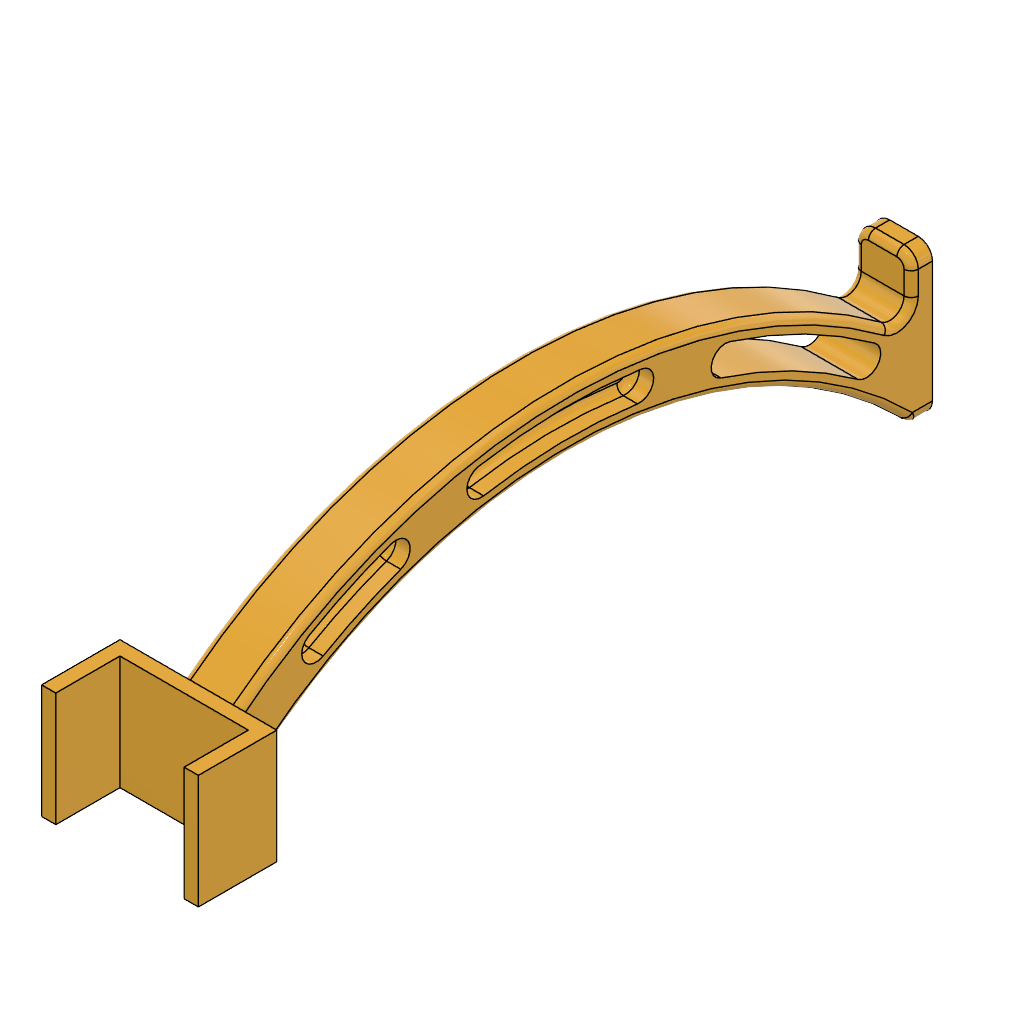
5. Marmik Shah_2026A4PS0775H - Landing Gear_Optimization study (Autodesk Fusion 360 design; units mm, degrees)
description: CATIA V5 STEP Exchange
part number: Landing stick.1.3
Autodesk Fusion 360 part; units mm, degrees
sketch "Sketch7" plane through (0, 0, 0) normal (0, 0, 1) x (1, 0, 0)
  line L0 (-11, 11) -> (11, 11)
  line L1 (11, 11) -> (11, -5)
  line L2 (11, -5) -> (-11, -5)
  line L3 (-11, -5) -> (-11, 11)
  dimension "d5" = 22
  dimension "d6" = 11
  dimension "d7" = 16
  dimension "d8" = 11
  constraint horizontal L0
  constraint vertical L1
  constraint horizontal L2
  constraint vertical L3
  measures "d5" distance of L0.start L0.end
  measures "d6" distance of origin L3
  measures "d7" distance of L0 L2
  measures "d8" distance of origin L0
extrude "Extrude1" add sketch "Sketch7" against normal blind 2
sketch "Sketch8" plane through (0, 0, 0) normal (1, 0, 0) x (0, 0, -1)
  arc A0 (98, 7.6281) -> (2, 7.6281) centre (50, -50) ccw
  arc A1 (98.7134, -4) -> (2, -3.256) centre (50, -50) ccw
  line L0 (98.7134, -4) -> (101, -4)
  line L1 (101, -4) -> (101, 17)
  line L2 (101, 17) -> (98, 17)
  line L3 (98, 17) -> (98, 7.6281)
  line L4 (2, -3.256) -> (2, 7.6281)
  dimension "d13" = 75
  dimension "d19" = 3
  dimension "d20" = 21
  dimension "d21" = 50
  dimension "d22" = 50
  dimension "d23" = 17
  dimension "d26" = 67
  dimension "d28" = 8
  dimension "d30" = 2
  dimension "d31" = 101
  constraint horizontal L0
  constraint vertical L1
  constraint horizontal L2
  constraint vertical L3
  constraint vertical A0.centre A1.centre
  constraint coincident A0.centre A1.centre
  constraint vertical L4
  measures "d13" radius of A0
  measures "d19" distance of L1 L3
  measures "d20" distance of L0.end L1.end
  measures "d21" horizontal distance of origin A0.centre
  measures "d22" vertical distance of origin A0.centre
  measures "d23" distance of origin L2
  measures "d26" radius of A1
  measures "d28" distance of A0 A1
  measures "d30" distance of origin L4
  measures "d31" distance of origin L1
extrude "Extrude3" add sketch "Sketch8" along normal blind 4 and the other way blind 4
sketch "Sketch11" plane through (0, 0, 0) normal (0, 0, 1) x (1, 0, 0)
  line L0 (-11, -5) -> (11, -5)
  line L1 (11, -5) -> (11, 11)
  line L2 (11, 11) -> (-11, 11)
  line L3 (-11, 11) -> (-11, -5)
  line L4 (11, -5) -> (9, -5)
  line L5 (9, -5) -> (9, 11)
  line L6 (9, 11) -> (11, 11)
  line L7 (11, 11) -> (11, -5)
  line L8 (-11, -5) -> (-9, -5)
  line L9 (-9, -5) -> (-9, 11)
  line L10 (-9, 11) -> (-11, 11)
  line L11 (-11, 11) -> (-11, -5)
  dimension "d84" = 2
  dimension "d85" = 2
  constraint coincident L0.start L3.end
  constraint horizontal L4
  constraint vertical L5
  constraint horizontal L6
  constraint vertical L7
  constraint horizontal L8
  constraint vertical L9
  constraint horizontal L10
  constraint vertical L11
  constraint horizontal L4.end L8.end
  constraint horizontal L5.end L9.end
  constraint coincident L2 L9.end
  constraint coincident L1.end L7
  measures "d84" distance of L5 L7
  measures "d85" distance of L9 L11
sketch "Sketch12" plane through (4, 0, 0) normal (1, 0, 0) x (0, 0, -1)
  line L0 (98.7134, -4) -> (101, -4)
  line L1 (101, -4) -> (101, 17)
  line L2 (101, 17) -> (98, 17)
  line L3 (98, 17) -> (98, 7.6281)
  arc A0 (98, 7.6281) -> (2, 7.6281) centre (50, -50) ccw
  line L4 (2, 7.6281) -> (2, -3.256)
  arc A1 (98.7134, -4) -> (2, -3.256) centre (50, -50) ccw
  arc A2 (98, 7.6281) -> (2, 7.6281) centre (50, -50) ccw
  arc A3 (25.0325, 18.5976) -> (13.5, 13.2199) centre (50, -50) ccw
  arc A4 (26.4006, 14.8388) -> (15.5, 9.7558) centre (50, -50) ccw
  arc A5 (13.5, 13.2199) -> (15.5, 9.7558) centre (14.5, 11.4878) ccw
  arc A6 (26.4006, 14.8388) -> (25.0325, 18.5976) centre (25.7166, 16.7182) ccw
  line L5 (50, -50) -> (14.5, 11.4878) construction
  line L6 (50, -50) -> (25.7166, 16.7182) construction
  line L7 (50, -50) -> (14.0011, -50) construction
  arc A7 (60.1596, 22.2896) -> (37.3237, 21.891) centre (50, -50) ccw
  arc A8 (59.6029, 18.3285) -> (38.0183, 17.9517) centre (50, -50) ccw
  arc A9 (37.3237, 21.891) -> (38.0183, 17.9517) centre (37.671, 19.9214) ccw
  arc A10 (59.6029, 18.3285) -> (60.1596, 22.2896) centre (59.8813, 20.309) ccw
  line L8 (50, -50) -> (37.671, 19.9214) construction
  line L9 (50, -50) -> (59.8813, 20.309) construction
  arc A11 (92.9083, 9.0582) -> (72.5582, 19.4271) centre (50, -50) ccw
  arc A12 (90.5572, 5.8222) -> (71.3222, 15.6229) centre (50, -50) ccw
  arc A13 (72.5582, 19.4271) -> (71.3222, 15.6229) centre (71.9402, 17.525) ccw
  arc A14 (90.5572, 5.8222) -> (92.9083, 9.0582) centre (91.7328, 7.4402) ccw
  line L10 (50, -50) -> (71.9402, 17.525) construction
  line L11 (50, -50) -> (91.7328, 7.4402) construction
  dimension "d46" = 73
  dimension "d47" = 4
  dimension "d48" = 2
  dimension "d49" = 2
  dimension "d50" = 10
  dimension "d51" = 60
  dimension "d54" = 73
  dimension "d55" = 4
  dimension "d56" = 2
  dimension "d57" = 2
  dimension "d58" = 18
  dimension "d59" = 10
  dimension "d60" = 73
  dimension "d61" = 4
  dimension "d62" = 2
  dimension "d63" = 2
  dimension "d64" = 18
  dimension "d65" = 10
  constraint coincident A0.centre A1.centre
  constraint tangent A3 A5
  constraint tangent A3 A6
  constraint coincident A5.centre L5.end
  constraint coincident A6.centre L6.end
  constraint horizontal L7
  constraint tangent A7 A9
  constraint tangent A7 A10
  constraint coincident A9.centre L8.end
  constraint coincident A10.centre L9.end
  constraint tangent A12 A13
  constraint tangent A12 A14
  constraint coincident A13.centre L10.end
  constraint coincident A14.centre L11.end
  measures "d46" radius of A3
  measures "d47" distance of A3 A4
  measures "d48" radius of A5
  measures "d49" radius of A6
  measures "d50" angle of L5 L6
  measures "d51" angle of L5 L7
  measures "d54" radius of A7
  measures "d55" distance of A7 A8
  measures "d56" radius of A10
  measures "d57" radius of A9
  measures "d58" angle of L8 L9
  measures "d59" angle of L6 L8
  measures "d60" radius of A11
  measures "d61" distance of A11 A12
  measures "d62" radius of A13
  measures "d63" radius of A14
  measures "d64" angle of L10 L11
  measures "d65" angle of L9 L10
extrude "Extrude5" cut sketch "Sketch12" against normal blind 3 contours A3 A4 A5 A6 | A7 A8 A9 A10
mirror "Mirror1" about plane through (0, 0, 0) normal (1, 0, 0) of "Extrude5"
fillet "Fillet6" radius 2 1 edges at (0, 7.6281, -98)
extrude "Extrude6" add sketch "Sketch11" along normal blind 9 contours L0 L2 L3 L8 L9 L10 L11 | L0 L1 L2 L4 L5 L6 L7
extrude "Extrude7" cut sketch "Sketch12" against normal up to surface (8 mm away) contours A11 A12 A13 A14
fillet "Fillet16" radius 2 4 edges at (4, 17, -99.5) (-4, 17, -99.5) (4, -4, -99.8567) (-4, -4, -99.8567)
fillet "Fillet17" radius 1 14 edges at (-4, 24.9724, -47.9663) (-4, 9.9621, -96.8973) (-4, 13.3747, -98) (-3.4142, 16.4142, -98) (0, 17, -98) (3.4142, 16.4142, -98) (4, 13.3747, -98) (4, 9.9621, -96.8973) (4, 24.9724, -47.9663) (4, 16.9941, -49.1119) (3.5199, -3.2996, -98.0424) (0, -4, -98.7134) (-3.5199, -3.2996, -98.0424) (-4, 16.9941, -49.1119)
fillet "Fillet18" radius 1 8 edges at (-3.7604, -2.7529, -2) (0, -3.256, -2) (3.7604, -2.7529, -2) (4, 2.2434, -2) (3.7497, 7.1858, -2) (0, 7.6281, -2) (-3.7497, 7.1858, -2) (-4, 2.2434, -2)
fillet "Fillet19" radius 1 8 edges at (1, 22.9889, -48.726) (1, 20.0307, -61.8618) (1, 18.9895, -48.7958) (1, 19.5741, -35.7014) (-1, 22.9889, -48.726) (-1, 20.0307, -61.8618) (-1, 18.9895, -48.7958) (-1, 19.5741, -35.7014)
fillet "Fillet20" radius 1 8 edges at (1, 16.1605, -19.1489) (1, 17.4022, -27.596) (1, 12.5352, -20.8393) (1, 10.4878, -12.7679) (-1, 10.4878, -12.7679) (-1, 16.1605, -19.1489) (-1, 17.4022, -27.596) (-1, 12.5352, -20.8393)
